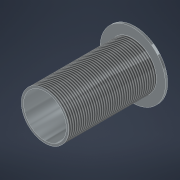
# Autodesk Inventor part: bearingShellInner
Saved by Autodesk Inventor 2021.4 (Build 254397000, 397)
## iProperties
Created: 2022-03-02
Part Number: bearingShellInner
Material: Generic
Document SubType Name: Modeling
Designer: jo_ki
Density: 1 g/cm^3
Appearance: Zinc
Author: jo_ki
Autodesk Inventor part; units mm, degrees
ref_plane "YZ Plane" through (0, 0, 0) normal (1, 0, 0) x (0, 1, 0)
ref_plane "XZ Plane" through (0, 0, 0) normal (0, 1, 0) x (-1, 0, 0)
ref_plane "XY Plane" through (0, 0, 0) normal (0, 0, 1) x (1, 0, 0)
sketch "Sketch1" plane through (0, 0, 0) normal (1, 0, 0) x (0, 1, 0)
  line L0 (10.5, -1) -> (9.5, -1)
  line L1 (9.5, -1) -> (9.5, -40)
  line L2 (9.5, -40) -> (10.5, -40)
  line L3 (10.5, -40) -> (10.5, -1)
  line L4 (14.5, -40) -> (8.5, -40)
  line L5 (8.5, -40) -> (8.5, -41)
  line L6 (8.5, -41) -> (14.5, -41)
  line L7 (14.5, -41) -> (14.5, -40)
  line L8 (0, -49.2) -> (0, 8.2) projected
  point P0 (0, 0)
  dimension "d0" = 1
  dimension "d1" = 1
  dimension "d2" = 1
  dimension "d3" = 10.5
  dimension "d4" = 4
  dimension "d5" = 40
  constraints: 16 end point, 4 parallel, 3 perpendicular, 2 horizontal, 1 point on line
  measures "d0" distance between parallel lines of L1 L5
  measures "d1" distance between parallel lines of L1 L3
  measures "d2" vertical distance of L0.end point (0, 0)
  measures "d3" distance from line of point (0, 0) L3
  measures "d4" distance from line of L3 L6.end
  measures "d5" distance from line of point (0, 0) L4
revolve "Revolution1" add sketch "Sketch1" angle 360 about axis through (0, 0, -10) along (0, 0, 1)
thread "Thread1" size "M22x1" class "6g" standard "ISO Metric profile" full length
body "Solid1"
